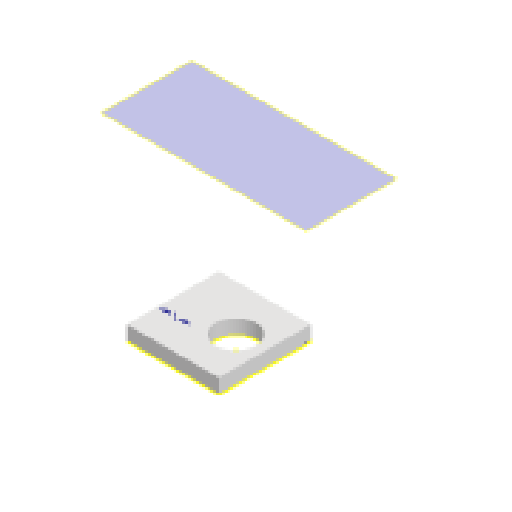
# Autodesk Inventor part: HolisheetCageSampleWater
Saved by Autodesk Inventor 2024.1 (Build 281209000, 209)
## iProperties
Created: 2024-08-13
Part Number: HolisheetCageSampleWater
Material: Generisch
Document SubType Name: Modeling
Designer: diederichbenedict
Density: 1 g/cm^3
Appearance: Vorgabe
Author: diederichbenedict
Autodesk Inventor part; units mm, degrees
ref_plane "YZ Plane" through (0, 0, 0) normal (1, 0, 0) x (0, 1, 0)
ref_plane "XZ Plane" through (0, 0, 0) normal (0, 1, 0) x (-1, 0, 0)
ref_plane "XY Plane" through (0, 0, 0) normal (0, 0, 1) x (1, 0, 0)
ref_plane "Arbeitsebene1" through (32.4682, 0, 46.5) normal (0, 0, -1) x (-1, 0, 0)
sketch "Skizze1" plane through (0, 0, 0) normal (0, 0, 1) x (1, 0, 0)
  circle A0 centre (0, 0) radius 4.1
  line L0 (-14.5, 14.5) -> (4.5, 14.5)
  line L1 (4.5, 14.5) -> (4.5, -4.5)
  line L2 (4.5, -4.5) -> (-14.5, -4.5)
  line L3 (-14.5, -4.5) -> (-14.5, 14.5)
  dimension "d0" = 8.2
  dimension "d1" = 19
  dimension "d2" = 19
  dimension "d3" = 4.5
  dimension "d4" = 4.5
  constraints: 8 end point, 2 parallel, 1 centre point, 1 coincident, 1 horizontal, 1 perpendicular
  measures "d0" diameter of A0
  measures "d1" distance of L1.end L2.end
  measures "d2" distance of L0.end L1.end
  measures "d3" distance from line of L2 point (0, 0)
  measures "d4" distance from line of L1 point (0, 0)
extrude "Extrusion1" add sketch "Skizze1" along normal blind 3
sketch "Skizze2" plane through (0, 0, 0) normal (0, 0, -1) x (-1, 0, 0)
  line L0 (14.5, 14.5) -> (14.5, -4.5) projected
  line L1 (-4.5, 14.5) -> (14.5, 14.5) projected
  circle A0 centre (0, 0) radius 4.1 projected
  line L2 (14.5, -4.5) -> (-4.5, -4.5) projected
  line L3 (-4.5, -4.5) -> (-4.5, 14.5) projected
  line L4 (-4.5, 14.5) -> (14.5, 14.5)
  line L5 (14.5, 14.5) -> (14.5, -4.5)
  line L6 (14.5, -4.5) -> (-4.5, -4.5)
  line L7 (-4.5, -4.5) -> (-4.5, 14.5)
  line L8 (-3, -4.5) -> (-3, 13)
  line L9 (-3, 13) -> (13, 13)
  line L10 (13, 13) -> (13, -3)
  line L11 (13, -3) -> (-0.4, -3)
  line L12 (-4.5, -4.5) -> (4.5, -4.5)
  line L13 (4.5, -4.5) -> (4.5, 4.5)
  line L14 (4.5, 4.5) -> (-4.5, 4.5)
  line L15 (-4.5, 4.5) -> (-4.5, -4.5)
  line L16 (-3, 13) -> (13, 13)
  line L17 (13, 13) -> (13, 14.5)
  line L18 (13, 14.5) -> (-3, 14.5)
  line L19 (-3, 14.5) -> (-3, 13)
  point P0 (4.5, -3)
  point P1 (4.5, -4.5)
  point P2 (13, 14.5)
  point P3 (-4.5, 4.5)
  point P4 (-3, 4.5)
  dimension "d13" = 1.5
  dimension "d14" = 9
  dimension "d15" = 9
  constraints: 32 end point, 6 parallel, 3 horizontal, 3 perpendicular, 1 point on line, 3 other
  measures "d13" distance between parallel lines of L3 L8
  measures "d14" distance of L14.end L13.end
  measures "d15" distance of L13.end L12.end
extrude "Extrusion2" add sketch "Skizze2" along normal blind 15 contours L0 L2 L13 L11 L10 L17 L1 | L19 L8 L14 L3 L1
sketch "Skizze3" plane through (0, 0, -15) normal (0, 0, -1) x (-1, 0, 0)
  line L0 (-4.5, 14.5) -> (14.5, 14.5) projected
  line L1 (14.5, 14.5) -> (14.5, -4.5) projected
  circle A0 centre (0, 0) radius 4.1 projected
  line L2 (14.5, -4.5) -> (-4.5, -4.5) projected
  line L3 (-4.5, -4.5) -> (-4.5, 14.5) projected
extrude "Extrusion3" add sketch "Skizze3" along normal blind 3
